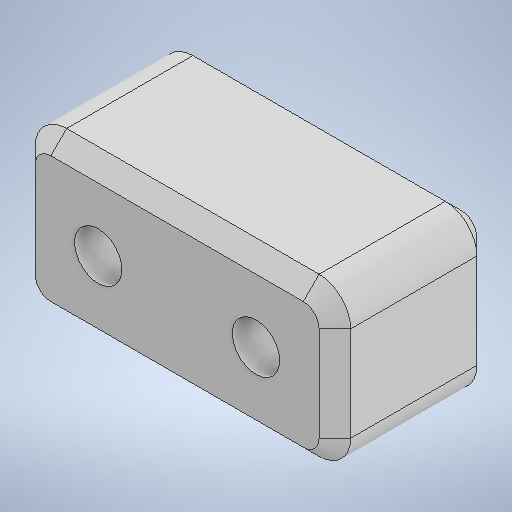
# Autodesk Inventor part: RobotBaseConnector1x2
Saved by Autodesk Inventor 2025.3 (Build 293356000, 356)
## iProperties
Created: 2025-04-28
Part Number: RobotBaseConnector1x2
Material: 일반
Document SubType Name: Modeling
Designer: SEON
Density: 1 g/cm^3
Appearance: 기본값
Author: SEON
Autodesk Inventor part; units mm, degrees
ref_plane "YZ Plane" through (0, 0, 0) normal (1, 0, 0) x (0, 1, 0)
ref_plane "XZ Plane" through (0, 0, 0) normal (0, 1, 0) x (-1, 0, 0)
ref_plane "XY Plane" through (0, 0, 0) normal (0, 0, 1) x (1, 0, 0)
sketch "스케치1" plane through (0, 0, 0) normal (0, 0, 1) x (1, 0, 0)
  line L0 (-10, -5) -> (10, -5)
  line L1 (10, -5) -> (10, 5)
  line L2 (10, 5) -> (-10, 5)
  line L3 (-10, 5) -> (-10, -5)
  line L4 (-10, -5) -> (10, 5) construction
  line L5 (10, -5) -> (-10, 5) construction
  circle A0 centre (-5, 0) radius 1.5
  circle A1 centre (5, 0) radius 1.5
  point P0 (0, 0)
  dimension "d0" = 10
  dimension "d1" = 20
  dimension "d2" = 3
  dimension "d3" = 5
  dimension "d4" = 5
  constraints: 12 end point, 2 centre point, 2 horizontal alignment, 2 midpoint, 2 parallel, 1 equal radius, 1 horizontal, 1 perpendicular
  measures "d0" distance of L2.end L0.start
  measures "d1" distance of L1.end L2.end
  measures "d2" diameter of A0
  measures "d3" distance from line of L3 A0.centre
  measures "d4" distance from line of L1 A1.centre
extrude "돌출1" add sketch "스케치1" along normal blind 10
fillet "모깎기1" radius 2 4 edges at (-10, 5, 5) (-10, -5, 5) (10, -5, 5) (10, 5, 5)
chamfer "모따기1" distance 1 angle 45 16 edges at (0, 5, 0) (-9.4142, 4.4142, 0) (-10, 0, 0) (-9.4142, -4.4142, 0) (0, -5, 0) (9.4142, -4.4142, 0) (10, 0, 0) (9.4142, 4.4142, 0) (0, 5, 10) (-9.4142, 4.4142, 10) (-10, 0, 10) (-9.4142, -4.4142, 10) (0, -5, 10) (9.4142, -4.4142, 10) (10, 0, 10) (9.4142, 4.4142, 10)
